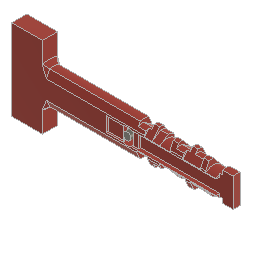
protec3 POC (Autodesk Fusion 360 design; units mm, degrees)
Autodesk Fusion 360 part; units mm, degrees
sketch "base/0 cut" plane through (0, 0, 0) normal (1, 0, 0) x (0, 1, 0)
  line L0 (0, 0) -> (3.3, 0)
  line L1 (3.3, 0) -> (3.3, 3.3)
  circle A0 centre (3.3, 3.3) radius 3.7125
  line L2 (3.3, 3.3) -> (4, 3.3)
  line L3 (3.3, 3.3) -> (2.6, 3.3)
  line L4 (4, 3.3) -> (4, 4.7)
  line L5 (4, 3.3) -> (4, 1.9)
  line L6 (2.6, 3.3) -> (2.6, 1.9)
  line L7 (2.6, 3.3) -> (2.6, 4.7)
  line L8 (4, 4.7) -> (4.775, 4.7)
  line L9 (4, 1.9) -> (4.775, 1.9)
  line L10 (2.6, 1.9) -> (1.825, 1.9)
  line L11 (2.6, 4.7) -> (1.825, 4.7)
  line L12 (4.775, 4.7) -> (4.775, 5.1226)
  line L13 (4.775, 1.9) -> (4.775, 1.4774)
  line L14 (1.825, 1.9) -> (1.825, 1.4774)
  line L15 (1.825, 4.7) -> (1.825, 5.1226)
  line L16 (4.775, 5.1226) -> (4.1363, 6.4923)
  line L17 (4.775, 5.1226) -> (1.825, 5.1226) construction
  line L18 (1.825, 5.1226) -> (2.4637, 6.4923)
  line L19 (1.825, 5.1226) -> (4.775, 5.1226) construction
  arc A1 (4.1363, 6.4923) -> (2.4637, 6.4923) centre (3.3, 3.3) ccw
  line L20 (4.775, 1.4774) -> (4.1363, 0.1077)
  line L21 (4.775, 1.4774) -> (1.825, 1.4774) construction
  line L22 (1.825, 1.4774) -> (2.4637, 0.1077)
  line L23 (1.825, 1.4774) -> (4.775, 1.4774) construction
  arc A2 (2.4637, 0.1077) -> (4.1363, 0.1077) centre (3.3, 3.3) ccw
  dimension "d27" = 3.3
  dimension "d28" = 3.3
  dimension "d29" = 7.425
  dimension "d30" = 0.7
  dimension "d31" = 0.7
  dimension "d32" = 1.4
  dimension "d33" = 1.4
  dimension "d34" = 1.4
  dimension "d35" = 1.4
  dimension "d36" = 0.775
  dimension "d37" = 0.775
  dimension "d38" = 0.775
  dimension "d39" = 0.775
  dimension "d40" = 0.4226
  dimension "d41" = 0.4226
  dimension "d42" = 0.4226
  dimension "d43" = 0.4226
  dimension "d44" = 65
  dimension "d45" = 1.5113
  dimension "d46" = 65
  dimension "d47" = 1.5113
  dimension "d48" = 65
  dimension "d49" = 1.5113
  dimension "d50" = 65
  dimension "d51" = 1.5113
  constraint coincident L0.start origin
  constraint horizontal L0
  constraint perpendicular L0 L1
  constraint coincident L1.end A0.centre
  constraint perpendicular L1 L2
  constraint perpendicular L1 L3
  constraint perpendicular L2 L4
  constraint perpendicular L2 L5
  constraint perpendicular L3 L6
  constraint perpendicular L3 L7
  constraint perpendicular L4 L8
  constraint perpendicular L5 L9
  constraint perpendicular L5 L10
  constraint perpendicular L7 L11
  constraint perpendicular L8 L12
  constraint perpendicular L9 L13
  constraint perpendicular L10 L14
  constraint perpendicular L11 L15
  constraint horizontal L17
  constraint horizontal L19
  constraint horizontal L21
  constraint horizontal L23
  measures "d27" distance of L0.start L0.end
  measures "d28" distance of L0.end L1.end
  measures "d29" diameter of A0
  measures "d30" distance of L1.end L2.end
  measures "d31" distance of L1.end L3.end
  measures "d32" distance of L2.end L4.end
  measures "d33" distance of L2.end L5.end
  measures "d34" distance of L3.end L6.end
  measures "d35" distance of L3.end L7.end
  measures "d36" distance of L4.end L8.end
  measures "d37" distance of L5.end L9.end
  measures "d38" distance of L6.end L10.end
  measures "d39" distance of L7.end L11.end
  measures "d40" distance of L8.end L12.end
  measures "d41" distance of L9.end L13.end
  measures "d42" distance of L10.end L14.end
  measures "d43" distance of L11.end L15.end
  measures "d44" angle of L16 L17
  measures "d45" distance of L12.end L16.end
  measures "d46" angle of L18 L19
  measures "d47" distance of L15.end L18.end
  measures "d48" angle of L20 L21
  measures "d49" distance of L13.end L20.end
  measures "d50" angle of L22 L23
  measures "d51" distance of L14.end L22.end
extrude "Extrude1" add sketch "base/0 cut" against normal blind 42.57 contours L1 L3 L6 L10 L14 L22 A2 | L1 L2 L5 L9 L13 L20 A2 | L2 L3 L4 L7 L8 L11 L12 L15 L16 L18 A1 makes body 1
sketch "bow and bearing retention" plane through (-42.57, 0, 0) normal (-1, 0, 0) x (0, -1, 0)
  line L0 (-2.6, 1.9) -> (-2.6, 4.7)
  line L1 (-2.6, 4.7) -> (-1.825, 4.7)
  line L2 (-1.825, 4.7) -> (-1.825, 5.1226)
  line L3 (-1.825, 5.1226) -> (-2.4637, 6.4923)
  arc A0 (-2.4637, 6.4923) -> (-4.1363, 6.4923) centre (-3.3, 3.3) ccw
  line L4 (-4.1363, 6.4923) -> (-4.775, 5.1226)
  line L5 (-4.775, 5.1226) -> (-4.775, 4.7)
  line L6 (-4.775, 4.7) -> (-4, 4.7)
  line L7 (-4, 4.7) -> (-4, 1.9)
  line L8 (-4, 1.9) -> (-4.775, 1.9)
  line L9 (-4.775, 1.9) -> (-4.775, 1.4774)
  line L10 (-4.775, 1.4774) -> (-4.1363, 0.1077)
  arc A1 (-4.1363, 0.1077) -> (-2.4637, 0.1077) centre (-3.3, 3.3) ccw
  line L11 (-2.4637, 0.1077) -> (-1.825, 1.4774)
  line L12 (-1.825, 1.4774) -> (-1.825, 1.9)
  line L13 (-1.825, 1.9) -> (-2.6, 1.9)
  line L14 (-2.6, 3.3) -> (-3.3, 3.3)
  line L15 (-3.3, 3.3) -> (-3.3, 6.6)
  circle A2 centre (-3.3, 3.3) radius 3.3
  line L16 (-4.775, 4.7) -> (-4.775, 6.252)
  line L17 (-4.775, 6.252) -> (-4.775, 11.252)
  line L18 (-1.825, 4.7) -> (-1.825, 6.252)
  line L19 (-1.825, 6.252) -> (-1.825, 11.252)
  line L20 (-4.775, 11.252) -> (-1.825, 11.252)
  line L21 (-1.825, 1.9) -> (-1.825, 0.348)
  line L22 (-1.825, 0.348) -> (-1.825, -4.652)
  line L23 (-4.775, 1.9) -> (-4.775, 0.348)
  line L24 (-4.775, 0.348) -> (-4.775, -4.652)
  line L25 (-4.775, -4.652) -> (-1.825, -4.652)
  line L26 (-4, 3.3) -> (-4.425, 3.3)
  line L27 (-4.425, 3.3) -> (-4.425, 4.7)
  line L28 (-4.425, 3.3) -> (-4.425, 1.9)
  line L29 (-2.6, 3.3) -> (-2.175, 3.3)
  line L30 (-2.175, 3.3) -> (-2.175, 1.9)
  line L31 (-2.175, 3.3) -> (-2.175, 4.7)
  line L32 (-1.825, 4.7) -> (-1.825, 1.9)
  line L33 (-4.775, 4.7) -> (-4.775, 1.9)
  dimension "d56" = 5
  dimension "d57" = 5
  dimension "d58" = 5
  dimension "d59" = 5
  dimension "d60" = 0.425
  dimension "d61" = 0.425
  constraint midpoint L0 L14.start
  constraint coincident A0.centre A1.centre
  constraint midpoint A0 L15.end
  constraint coincident L15.end A2
  constraint coincident L5.end L6.start
  constraint coincident A2 L16.end
  constraint perpendicular L6 L16
  constraint parallel L16 L17
  constraint coincident L1.end L2.start
  constraint coincident A2 L18.end
  constraint perpendicular L1 L18
  constraint parallel L18 L19
  constraint coincident L12.end L13.start
  constraint coincident A2 L21.end
  constraint perpendicular L13 L21
  constraint parallel L21 L22
  constraint coincident L8.end L9.start
  constraint coincident A2 L23.end
  constraint perpendicular L8 L23
  constraint parallel L23 L24
  constraint midpoint L7 L26.start
  constraint perpendicular L7 L26
  constraint coincident L6 L27.end
  constraint perpendicular L6 L27
  constraint coincident L8 L28.end
  constraint perpendicular L8 L28
  constraint perpendicular L0 L29
  constraint coincident L13 L30.end
  constraint perpendicular L13 L30
  constraint coincident L1 L31.end
  constraint perpendicular L1 L31
  measures "d56" distance of L16.end L17.end
  measures "d57" distance of L18.end L19.end
  measures "d58" distance of L21.end L22.end
  measures "d59" distance of L23.end L24.end
  measures "d60" distance of L26.start L26.end
  measures "d61" distance of L14.start L29.end
extrude "making bearing area wider" add sketch "bow and bearing retention" against normal blind 25.625 contours L0 L13 L29 L30 | L0 L1 L29 L31 | L6 L7 L26 L27 | L7 L8 L26 L28 bodies 1
extrude "making bow" add sketch "bow and bearing retention" against normal blind 6 contours L0 A0 L4 L5 L6 L7 L8 L9 L10 A1 L11 L12 L13 L14 L15 A2 L16 L21 L23 | L0 L13 L29 L30 | L0 L1 L2 L3 A0 L14 L15 A2 L18 | L0 L1 L29 L31 | L1 L13 L30 L31 L32 | A0 A2 L17 L19 L20 | L11 A2 L21 | L3 A2 L18 | L4 A2 L16 | A1 A2 L22 L24 L25 | L10 A2 L23 | L6 L8 L27 L28 L33 | L6 L7 L26 L27 | L7 L8 L26 L28 bodies 1
extrude "strengthening shaft" add 2 faces at (-36.57, 1.9417, 2.8333) (-36.57, 4.5417, 3.7667) along direction (1, 0, 0) blind 12.5 on bodies 1 bodies 1
chamfer "Chamfer1" distance 0.8 angle 45 6 edges at (-36.57, 3.3, 6.6) (-36.57, 2.1443, 5.8074) (-36.57, 4.4557, 5.8074) (-36.57, 4.4557, 0.7926) (-36.57, 3.3, 0) (-36.57, 2.1443, 0.7926) on bodies 1
sketch "tip cut" plane through (0, 0, 0) normal (1, 0, 0) x (0, 1, 0)
  line L0 (0, 0) -> (3.3, 0)
  line L1 (3.3, 0) -> (3.3, 3.3)
  line L2 (3.3, 3.3) -> (2.6, 3.3)
  line L3 (3.3, 3.3) -> (4, 3.3)
  circle A0 centre (3.3, 3.3) radius 2.9
  circle A1 centre (3.3, 3.3) radius 3.3
  line L4 (4, 3.3) -> (4, 0.4858)
  line L5 (4, 3.3) -> (4, 6.1142)
  line L6 (2.6, 3.3) -> (2.6, 0.4858)
  line L7 (2.6, 3.3) -> (2.6, 6.1142)
  dimension "d98" = 3.3
  dimension "d99" = 3.3
  dimension "d100" = 0.7
  dimension "d101" = 0.7
  dimension "d102" = 5.8
  dimension "d103" = 6.6
  constraint coincident L0.start origin
  constraint horizontal L0
  constraint perpendicular L0 L1
  constraint perpendicular L1 L2
  constraint perpendicular L1 L3
  constraint coincident L1.end L2.start
  constraint concentric A0 A1
  constraint coincident A0 L4.end
  constraint perpendicular L3 L4
  constraint coincident A0 L5.end
  constraint perpendicular L3 L5
  constraint coincident A0 L6.end
  constraint perpendicular L2 L6
  constraint coincident A0 L7.end
  constraint perpendicular L2 L7
  measures "d98" distance of L0.start L0.end
  measures "d99" distance of L0.end L1.end
  measures "d100" distance of L1.end L2.end
  measures "d101" distance of L1.end L3.end
  measures "d102" diameter of A0
  measures "d103" diameter of A1
sketch "1 cut" plane through (0, 0, 0) normal (1, 0, 0) x (0, 1, 0)
  line L0 (0, 0) -> (3.3, 0)
  line L1 (3.3, 0) -> (3.3, 3.3)
  line L2 (3.3, 3.3) -> (4, 3.3)
  line L3 (3.3, 3.3) -> (2.6, 3.3)
  line L4 (4, 3.3) -> (4, 4.7)
  line L5 (4, 3.3) -> (4, 1.9)
  line L6 (2.6, 3.3) -> (2.6, 1.9)
  line L7 (2.6, 3.3) -> (2.6, 4.7)
  line L8 (4, 4.7) -> (4.775, 4.7)
  line L9 (4, 1.9) -> (4.775, 1.9)
  line L10 (2.6, 1.9) -> (1.825, 1.9)
  line L11 (2.6, 4.7) -> (1.825, 4.7)
  line L12 (4.775, 4.7) -> (4.775, 4.8422)
  line L13 (1.825, 1.9) -> (1.825, 1.7578)
  line L14 (1.825, 4.7) -> (1.825, 5.1226)
  line L15 (4.775, 1.9) -> (4.775, 1.4774)
  line L16 (1.825, 5.1226) -> (2.4637, 6.4923)
  line L17 (1.825, 5.1226) -> (4.5397, 5.1226) construction
  line L18 (4.775, 1.4774) -> (4.1363, 0.1077)
  line L19 (4.775, 1.4774) -> (2.0603, 1.4774) construction
  line L20 (1.825, 1.7578) -> (3.3, 0)
  line L21 (1.825, 1.7578) -> (4.775, 1.7578) construction
  line L22 (4.775, 4.8422) -> (3.3, 6.6)
  line L23 (4.775, 4.8422) -> (1.825, 4.8422) construction
  arc A0 (3.3, 6.6) -> (2.4637, 6.4923) centre (3.3, 3.3) ccw
  arc A1 (3.3, 0) -> (4.1363, 0.1077) centre (3.3, 3.3) ccw
  circle A2 centre (3.3, 3.3) radius 3.7125
  dimension "d104" = 3.3
  dimension "d105" = 3.3
  dimension "d106" = 0.7
  dimension "d107" = 0.7
  dimension "d108" = 1.4
  dimension "d109" = 1.4
  dimension "d110" = 1.4
  dimension "d111" = 1.4
  dimension "d112" = 0.775
  dimension "d113" = 0.775
  dimension "d114" = 0.775
  dimension "d115" = 0.775
  dimension "d116" = 0.1422
  dimension "d117" = 0.1422
  dimension "d118" = 0.4226
  dimension "d119" = 0.4226
  dimension "d120" = 65
  dimension "d121" = 1.5113
  dimension "d122" = 65
  dimension "d123" = 1.5113
  dimension "d124" = 50
  dimension "d125" = 2.2947
  dimension "d126" = 50
  dimension "d127" = 2.2947
  dimension "d128" = 3.3
  dimension "d129" = 3.3
  dimension "d130" = 7.425
  constraint coincident L0.start origin
  constraint horizontal L0
  constraint perpendicular L0 L1
  constraint perpendicular L1 L2
  constraint perpendicular L1 L3
  constraint perpendicular L2 L4
  constraint perpendicular L2 L5
  constraint perpendicular L3 L6
  constraint perpendicular L3 L7
  constraint perpendicular L4 L8
  constraint perpendicular L5 L9
  constraint perpendicular L6 L10
  constraint perpendicular L7 L11
  constraint perpendicular L8 L12
  constraint perpendicular L10 L13
  constraint perpendicular L11 L14
  constraint perpendicular L9 L15
  constraint horizontal L17
  constraint horizontal L19
  constraint horizontal L21
  constraint horizontal L23
  constraint coincident L14 L23.end
  constraint coincident L17.end L22
  constraint coincident L15 L21.end
  constraint coincident L19.end L20
  constraint concentric A0 A2
  measures "d104" distance of L0.start L0.end
  measures "d105" distance of L0.end L1.end
  measures "d106" distance of L1.end L2.end
  measures "d107" distance of L1.end L3.end
  measures "d108" distance of L2.end L4.end
  measures "d109" distance of L2.end L5.end
  measures "d110" distance of L3.end L6.end
  measures "d111" distance of L3.end L7.end
  measures "d112" distance of L4.end L8.end
  measures "d113" distance of L5.end L9.end
  measures "d114" distance of L6.end L10.end
  measures "d115" distance of L7.end L11.end
  measures "d116" distance of L8.end L12.end
  measures "d117" distance of L10.end L13.end
  measures "d118" distance of L11.end L14.end
  measures "d119" distance of L9.end L15.end
  measures "d120" angle of L16 L17
  measures "d121" distance of L14.end L16.end
  measures "d122" angle of L18 L19
  measures "d123" distance of L15.end L18.end
  measures "d124" angle of L20 L21
  measures "d125" distance of L13.end L0.end
  measures "d126" angle of L22 L23
  measures "d127" distance of L12.end L22.end
  measures "d128" radius of A0
  measures "d129" radius of A1
  measures "d130" diameter of A2
sketch "2 cut" plane through (0, 0, 0) normal (1, 0, 0) x (0, 1, 0)
  line L0 (0, 0) -> (3.3, 0)
  line L1 (3.3, 0) -> (3.3, 3.3)
  line L2 (3.3, 3.3) -> (4, 3.3)
  line L3 (3.3, 3.3) -> (2.6, 3.3)
  line L4 (4, 3.3) -> (4, 4.7)
  line L5 (4, 3.3) -> (4, 1.9)
  line L6 (2.6, 3.3) -> (2.6, 1.9)
  line L7 (2.6, 3.3) -> (2.6, 4.7)
  line L8 (4, 4.7) -> (4.775, 4.7)
  line L9 (4, 1.9) -> (4.775, 1.9)
  line L10 (2.6, 1.9) -> (1.825, 1.9)
  line L11 (2.6, 4.7) -> (1.825, 4.7)
  line L12 (1.825, 4.7) -> (1.825, 4.8422)
  line L13 (4.775, 1.9) -> (4.775, 1.7578)
  line L14 (4.775, 4.7) -> (4.775, 5.1226)
  line L15 (1.825, 1.9) -> (1.825, 1.4774)
  line L16 (1.825, 1.4774) -> (2.4637, 0.1077)
  line L17 (1.825, 1.4774) -> (4.5397, 1.4774) construction
  line L18 (4.775, 5.1226) -> (4.1363, 6.4923)
  line L19 (4.775, 5.1226) -> (2.0603, 5.1226) construction
  line L20 (1.825, 4.8422) -> (3.3, 6.6)
  line L21 (1.825, 4.8422) -> (4.775, 4.8422) construction
  line L22 (4.775, 1.7578) -> (3.3, 0)
  line L23 (4.775, 1.7578) -> (1.825, 1.7578) construction
  arc A0 (2.4637, 0.1077) -> (3.3, 0) centre (3.3, 3.3) ccw
  arc A1 (4.1363, 6.4923) -> (3.3, 6.6) centre (3.3, 3.3) ccw
  circle A2 centre (3.3, 3.3) radius 3.7125
  dimension "d131" = 3.3
  dimension "d132" = 3.3
  dimension "d133" = 0.7
  dimension "d134" = 0.7
  dimension "d135" = 1.4
  dimension "d136" = 1.4
  dimension "d137" = 1.4
  dimension "d138" = 1.4
  dimension "d139" = 0.775
  dimension "d140" = 0.775
  dimension "d141" = 0.775
  dimension "d142" = 0.775
  dimension "d143" = 0.1422
  dimension "d144" = 0.1422
  dimension "d145" = 0.4226
  dimension "d146" = 0.4226
  dimension "d147" = 65
  dimension "d148" = 1.5113
  dimension "d149" = 65
  dimension "d150" = 1.5113
  dimension "d151" = 50
  dimension "d152" = 2.2947
  dimension "d153" = 50
  dimension "d154" = 2.2947
  dimension "d155" = 3.3
  dimension "d156" = 3.3
  dimension "d157" = 7.425
  constraint coincident L0.start origin
  constraint horizontal L0
  constraint perpendicular L0 L1
  constraint perpendicular L1 L2
  constraint perpendicular L1 L3
  constraint perpendicular L2 L4
  constraint perpendicular L2 L5
  constraint perpendicular L3 L6
  constraint perpendicular L3 L7
  constraint perpendicular L4 L8
  constraint perpendicular L5 L9
  constraint perpendicular L6 L10
  constraint perpendicular L7 L11
  constraint perpendicular L11 L12
  constraint perpendicular L9 L13
  constraint perpendicular L8 L14
  constraint perpendicular L10 L15
  constraint horizontal L17
  constraint horizontal L19
  constraint horizontal L21
  constraint horizontal L23
  constraint concentric A1 A2
  constraint coincident L15 L23.end
  constraint coincident L17.end L22
  constraint coincident L14 L21.end
  constraint coincident L19.end L20
  measures "d131" distance of L0.start L0.end
  measures "d132" distance of L0.end L1.end
  measures "d133" distance of L1.end L2.end
  measures "d134" distance of L1.end L3.end
  measures "d135" distance of L2.end L4.end
  measures "d136" distance of L2.end L5.end
  measures "d137" distance of L3.end L6.end
  measures "d138" distance of L3.end L7.end
  measures "d139" distance of L4.end L8.end
  measures "d140" distance of L5.end L9.end
  measures "d141" distance of L6.end L10.end
  measures "d142" distance of L7.end L11.end
  measures "d143" distance of L11.end L12.end
  measures "d144" distance of L9.end L13.end
  measures "d145" distance of L8.end L14.end
  measures "d146" distance of L10.end L15.end
  measures "d147" angle of L16 L17
  measures "d148" distance of L15.end L16.end
  measures "d149" angle of L18 L19
  measures "d150" distance of L14.end L18.end
  measures "d151" angle of L20 L21
  measures "d152" distance of L12.end L20.end
  measures "d153" angle of L22 L23
  measures "d154" distance of L13.end L0.end
  measures "d155" radius of A0
  measures "d156" radius of A1
  measures "d157" diameter of A2
sketch "3 cut" plane through (0, 0, 0) normal (1, 0, 0) x (0, 1, 0)
  line L0 (0, 0) -> (3.3, 0)
  line L1 (3.3, 0) -> (3.3, 3.3)
  line L2 (3.3, 3.3) -> (4, 3.3)
  line L3 (3.3, 3.3) -> (2.6, 3.3)
  line L4 (4, 3.3) -> (4, 4.7)
  line L5 (4, 3.3) -> (4, 1.9)
  line L6 (2.6, 3.3) -> (2.6, 1.9)
  line L7 (2.6, 3.3) -> (2.6, 4.7)
  line L8 (4, 4.7) -> (4.775, 4.7)
  line L9 (4, 1.9) -> (4.775, 1.9)
  line L10 (2.6, 1.9) -> (1.825, 1.9)
  line L11 (2.6, 4.7) -> (1.825, 4.7)
  line L12 (4.775, 4.7) -> (4.775, 4.8422)
  line L13 (1.825, 1.9) -> (1.825, 1.7578)
  line L14 (1.825, 4.7) -> (1.825, 5.1226)
  line L15 (4.775, 1.9) -> (4.775, 1.4774)
  line L16 (4.775, 1.4774) -> (4.4962, 0.8794)
  line L17 (4.775, 1.4774) -> (2.2255, 1.4774) construction
  line L18 (1.825, 5.1226) -> (2.1038, 5.7206)
  line L19 (1.825, 5.1226) -> (4.3745, 5.1226) construction
  line L20 (4.775, 4.8422) -> (3.1292, 5.9946)
  line L21 (4.775, 4.8422) -> (1.825, 4.8422) construction
  line L22 (1.825, 1.7578) -> (3.4708, 0.6054)
  line L23 (1.825, 1.7578) -> (4.775, 1.7578) construction
  arc A0 (3.1292, 5.9946) -> (2.1038, 5.7206) centre (3.3, 3.3) ccw
  arc A1 (3.4708, 0.6054) -> (4.4962, 0.8794) centre (3.3, 3.3) ccw
  circle A2 centre (3.3, 3.3) radius 3.7125
  dimension "d158" = 3.3
  dimension "d159" = 3.3
  dimension "d160" = 0.7
  dimension "d161" = 0.7
  dimension "d162" = 1.4
  dimension "d163" = 1.4
  dimension "d164" = 1.4
  dimension "d165" = 1.4
  dimension "d166" = 0.775
  dimension "d167" = 0.775
  dimension "d168" = 0.775
  dimension "d169" = 0.775
  dimension "d170" = 0.1422
  dimension "d171" = 0.1422
  dimension "d172" = 0.4226
  dimension "d173" = 0.4226
  dimension "d174" = 65
  dimension "d175" = 0.6598
  dimension "d176" = 65
  dimension "d177" = 0.6598
  dimension "d178" = 35
  dimension "d179" = 2.0092
  dimension "d180" = 35
  dimension "d181" = 2.0092
  dimension "d182" = 2.7
  dimension "d183" = 2.7
  dimension "d184" = 7.425
  constraint coincident L0.start origin
  constraint horizontal L0
  constraint perpendicular L0 L1
  constraint perpendicular L1 L2
  constraint perpendicular L1 L3
  constraint perpendicular L2 L4
  constraint perpendicular L2 L5
  constraint perpendicular L3 L6
  constraint perpendicular L3 L7
  constraint perpendicular L4 L8
  constraint perpendicular L5 L9
  constraint perpendicular L6 L10
  constraint perpendicular L7 L11
  constraint perpendicular L8 L12
  constraint perpendicular L10 L13
  constraint perpendicular L11 L14
  constraint perpendicular L9 L15
  constraint horizontal L17
  constraint horizontal L19
  constraint horizontal L21
  constraint horizontal L23
  constraint coincident L17.end L22
  constraint coincident L14 L21.end
  constraint coincident L19.end L20
  constraint coincident L15 L23.end
  constraint concentric A0 A2
  measures "d158" distance of L0.start L0.end
  measures "d159" distance of L0.end L1.end
  measures "d160" distance of L1.end L2.end
  measures "d161" distance of L1.end L3.end
  measures "d162" distance of L2.end L4.end
  measures "d163" distance of L2.end L5.end
  measures "d164" distance of L3.end L6.end
  measures "d165" distance of L3.end L7.end
  measures "d166" distance of L4.end L8.end
  measures "d167" distance of L5.end L9.end
  measures "d168" distance of L6.end L10.end
  measures "d169" distance of L7.end L11.end
  measures "d170" distance of L8.end L12.end
  measures "d171" distance of L10.end L13.end
  measures "d172" distance of L11.end L14.end
  measures "d173" distance of L9.end L15.end
  measures "d174" angle of L16 L17
  measures "d175" distance of L15.end L16.end
  measures "d176" angle of L18 L19
  measures "d177" distance of L14.end L18.end
  measures "d178" angle of L20 L21
  measures "d179" distance of L12.end L20.end
  measures "d180" angle of L22 L23
  measures "d181" distance of L13.end L22.end
  measures "d182" radius of A0
  measures "d183" radius of A1
  measures "d184" diameter of A2
sketch "4 cut" plane through (0, 0, 0) normal (1, 0, 0) x (0, 1, 0)
  line L0 (0, 0) -> (3.3, 0)
  line L1 (3.3, 0) -> (3.3, 3.3)
  line L2 (3.3, 3.3) -> (4, 3.3)
  line L3 (3.3, 3.3) -> (2.6, 3.3)
  line L4 (4, 3.3) -> (4, 1.9)
  line L5 (4, 3.3) -> (4, 4.7)
  line L6 (2.6, 3.3) -> (2.6, 1.9)
  line L7 (2.6, 3.3) -> (2.6, 4.7)
  line L8 (4, 4.7) -> (4.775, 4.7)
  line L9 (4, 1.9) -> (4.775, 1.9)
  line L10 (2.6, 1.9) -> (1.825, 1.9)
  line L11 (2.6, 4.7) -> (1.825, 4.7)
  line L12 (4.775, 4.7) -> (4.775, 4.8422)
  line L13 (1.825, 4.7) -> (1.825, 4.8422)
  line L14 (4.775, 1.9) -> (4.775, 1.7578)
  line L15 (1.825, 1.9) -> (1.825, 1.7578)
  line L16 (4.775, 4.8422) -> (3.8512, 5.9431)
  line L17 (4.775, 4.8422) -> (1.825, 4.8422) construction
  line L18 (1.825, 4.8422) -> (2.7488, 5.9431)
  line L19 (1.825, 4.8422) -> (4.775, 4.8422) construction
  line L20 (4.775, 1.7578) -> (3.8512, 0.6569)
  line L21 (4.775, 1.7578) -> (1.825, 1.7578) construction
  line L22 (1.825, 1.7578) -> (2.7488, 0.6569)
  line L23 (1.825, 1.7578) -> (4.775, 1.7578) construction
  arc A0 (3.8512, 5.9431) -> (2.7488, 5.9431) centre (3.3, 3.3) ccw
  arc A1 (2.7488, 0.6569) -> (3.8512, 0.6569) centre (3.3, 3.3) ccw
  circle A2 centre (3.3, 3.3) radius 3.7125
  dimension "d185" = 3.3
  dimension "d186" = 3.3
  dimension "d187" = 0.7
  dimension "d188" = 0.7
  dimension "d189" = 1.4
  dimension "d190" = 1.4
  dimension "d191" = 1.4
  dimension "d192" = 1.4
  dimension "d193" = 0.775
  dimension "d194" = 0.775
  dimension "d195" = 0.775
  dimension "d196" = 0.775
  dimension "d197" = 0.1422
  dimension "d198" = 0.1422
  dimension "d199" = 0.1422
  dimension "d200" = 0.1422
  dimension "d201" = 50
  dimension "d202" = 1.4372
  dimension "d203" = 50
  dimension "d204" = 1.4372
  dimension "d205" = 50
  dimension "d206" = 1.4372
  dimension "d207" = 50
  dimension "d208" = 1.4372
  dimension "d209" = 7.425
  constraint coincident L0.start origin
  constraint horizontal L0
  constraint perpendicular L0 L1
  constraint perpendicular L1 L2
  constraint perpendicular L1 L3
  constraint perpendicular L3 L4
  constraint perpendicular L2 L5
  constraint perpendicular L3 L6
  constraint perpendicular L3 L7
  constraint perpendicular L5 L8
  constraint perpendicular L4 L9
  constraint perpendicular L6 L10
  constraint perpendicular L7 L11
  constraint perpendicular L8 L12
  constraint perpendicular L11 L13
  constraint perpendicular L9 L14
  constraint perpendicular L10 L15
  constraint horizontal L17
  constraint horizontal L19
  constraint horizontal L21
  constraint horizontal L23
  constraint coincident L1.end L2.start
  constraint concentric A0 A2
  measures "d185" distance of L0.start L0.end
  measures "d186" distance of L0.end L1.end
  measures "d187" distance of L1.end L2.end
  measures "d188" distance of L1.end L3.end
  measures "d189" distance of L2.end L4.end
  measures "d190" distance of L2.end L5.end
  measures "d191" distance of L3.end L6.end
  measures "d192" distance of L3.end L7.end
  measures "d193" distance of L5.end L8.end
  measures "d194" distance of L4.end L9.end
  measures "d195" distance of L6.end L10.end
  measures "d196" distance of L7.end L11.end
  measures "d197" distance of L8.end L12.end
  measures "d198" distance of L11.end L13.end
  measures "d199" distance of L9.end L14.end
  measures "d200" distance of L10.end L15.end
  measures "d201" angle of L16 L17
  measures "d202" distance of L12.end L16.end
  measures "d203" angle of L18 L19
  measures "d204" distance of L13.end L18.end
  measures "d205" angle of L20 L21
  measures "d206" distance of L14.end L20.end
  measures "d207" angle of L22 L23
  measures "d208" distance of L15.end L22.end
  measures "d209" diameter of A2
sketch "5 cut" plane through (0, 0, 0) normal (1, 0, 0) x (0, 1, 0)
  line L0 (0, 0) -> (3.3, 0)
  line L1 (3.3, 0) -> (3.3, 3.3)
  line L2 (3.3, 3.3) -> (4, 3.3)
  line L3 (3.3, 3.3) -> (2.6, 3.3)
  line L4 (4, 3.3) -> (4, 4.7)
  line L5 (4, 3.3) -> (4, 1.9)
  line L6 (2.6, 3.3) -> (2.6, 1.9)
  line L7 (2.6, 3.3) -> (2.6, 4.7)
  line L8 (4, 4.7) -> (4.775, 4.7)
  line L9 (4, 1.9) -> (4.775, 1.9)
  line L10 (2.6, 1.9) -> (1.825, 1.9)
  line L11 (2.6, 4.7) -> (1.825, 4.7)
  line L12 (1.825, 4.7) -> (1.825, 4.8422)
  line L13 (4.775, 1.9) -> (4.775, 1.7578)
  line L14 (1.825, 1.9) -> (1.825, 1.4774)
  line L15 (4.775, 4.7) -> (4.775, 5.1226)
  line L16 (1.825, 4.8422) -> (3.4708, 5.9946)
  line L17 (1.825, 4.8422) -> (4.775, 4.8422) construction
  line L18 (4.775, 1.7578) -> (3.1292, 0.6054)
  line L19 (4.775, 1.7578) -> (1.825, 1.7578) construction
  line L20 (1.825, 1.4774) -> (2.1038, 0.8794)
  line L21 (1.825, 1.4774) -> (4.3745, 1.4774) construction
  line L22 (4.775, 5.1226) -> (4.4962, 5.7206)
  line L23 (4.775, 5.1226) -> (2.2255, 5.1226) construction
  arc A0 (4.4962, 5.7206) -> (3.4708, 5.9946) centre (3.3, 3.3) ccw
  arc A1 (2.1038, 0.8794) -> (3.1292, 0.6054) centre (3.3, 3.3) ccw
  circle A2 centre (3.3, 3.3) radius 3.7125
  dimension "d210" = 3.3
  dimension "d211" = 3.3
  dimension "d212" = 0.7
  dimension "d213" = 0.7
  dimension "d214" = 1.4
  dimension "d215" = 1.4
  dimension "d216" = 1.4
  dimension "d217" = 1.4
  dimension "d218" = 0.775
  dimension "d219" = 0.775
  dimension "d220" = 0.775
  dimension "d221" = 0.775
  dimension "d222" = 0.1422
  dimension "d223" = 0.1422
  dimension "d224" = 0.4226
  dimension "d225" = 0.4226
  dimension "d226" = 35
  dimension "d227" = 2.0092
  dimension "d228" = 35
  dimension "d229" = 2.0092
  dimension "d230" = 0.6598
  dimension "d231" = 65
  dimension "d232" = 65
  dimension "d233" = 0.6598
  dimension "d234" = 2.7
  dimension "d235" = 2.7
  dimension "d236" = 7.425
  constraint coincident L0.start origin
  constraint horizontal L0
  constraint perpendicular L0 L1
  constraint perpendicular L1 L2
  constraint perpendicular L1 L3
  constraint perpendicular L2 L4
  constraint perpendicular L2 L5
  constraint perpendicular L3 L6
  constraint perpendicular L3 L7
  constraint perpendicular L4 L8
  constraint perpendicular L5 L9
  constraint perpendicular L6 L10
  constraint perpendicular L7 L11
  constraint perpendicular L11 L12
  constraint perpendicular L9 L13
  constraint perpendicular L10 L14
  constraint perpendicular L8 L15
  constraint horizontal L17
  constraint horizontal L19
  constraint horizontal L21
  constraint horizontal L23
  constraint concentric A0 A2
  constraint coincident L14 L19.end
  constraint coincident L18 L21.end
  constraint coincident L15 L17.end
  constraint coincident L16 L23.end
  measures "d210" distance of L0.start L0.end
  measures "d211" distance of L0.end L1.end
  measures "d212" distance of L1.end L2.end
  measures "d213" distance of L1.end L3.end
  measures "d214" distance of L2.end L4.end
  measures "d215" distance of L2.end L5.end
  measures "d216" distance of L3.end L6.end
  measures "d217" distance of L3.end L7.end
  measures "d218" distance of L4.end L8.end
  measures "d219" distance of L5.end L9.end
  measures "d220" distance of L6.end L10.end
  measures "d221" distance of L7.end L11.end
  measures "d222" distance of L11.end L12.end
  measures "d223" distance of L9.end L13.end
  measures "d224" distance of L10.end L14.end
  measures "d225" distance of L8.end L15.end
  measures "d226" angle of L16 L17
  measures "d227" distance of L12.end L16.end
  measures "d228" angle of L18 L19
  measures "d229" distance of L13.end L18.end
  measures "d230" distance of L14.end L20.end
  measures "d231" angle of L20 L21
  measures "d232" angle of L22 L23
  measures "d233" distance of L15.end L22.end
  measures "d234" radius of A0
  measures "d235" radius of A1
  measures "d236" diameter of A2
sketch "6 cut" plane through (0, 0, 0) normal (1, 0, 0) x (0, 1, 0)
  line L0 (0, 0) -> (3.3, 0)
  line L1 (3.3, 0) -> (3.3, 3.3)
  line L2 (3.3, 3.3) -> (4, 3.3)
  line L3 (4, 3.3) -> (4, 4.7)
  line L4 (4, 4.7) -> (4.775, 4.7)
  line L5 (4.775, 4.7) -> (4.775, 4.8422)
  line L6 (4.775, 4.8422) -> (3.1292, 5.9946) construction
  line L7 (4.775, 4.8422) -> (1.861, 4.8422) construction
  circle A0 centre (3.3, 3.3) radius 2.1093
  circle A1 centre (3.3, 3.3) radius 3.7125
  dimension "d237" = 3.3
  dimension "d238" = 3.3
  dimension "d239" = 0.7
  dimension "d240" = 1.4
  dimension "d241" = 0.775
  dimension "d242" = 0.1422
  dimension "d243" = 35
  dimension "d244" = 2.0092
  dimension "d245" = 7.425
  constraint coincident L0.start origin
  constraint horizontal L0
  constraint perpendicular L0 L1
  constraint perpendicular L1 L2
  constraint perpendicular L2 L3
  constraint perpendicular L3 L4
  constraint perpendicular L4 L5
  constraint horizontal L7
  constraint coincident L1.end L2.start
  constraint tangent L6 A0
  constraint coincident L7.end A0
  constraint concentric A0 A1
  measures "d237" distance of L0.start L0.end
  measures "d238" distance of L0.end L1.end
  measures "d239" distance of L1.end L2.end
  measures "d240" distance of L2.end L3.end
  measures "d241" distance of L3.end L4.end
  measures "d242" distance of L4.end L5.end
  measures "d243" angle of L6 L7
  measures "d244" distance of L5.end L6.end
  measures "d245" diameter of A1
extrude "tip" cut sketch "tip cut" against normal blind 2.57 contours A0 L6 L7 | A0 L4 L5 | A1 bodies 1
extrude "0" cut sketch "6 cut" along normal mid plane 1 from surface at -2.57 bodies 1
extrude "1" cut sketch "6 cut" along normal mid plane 2 from surface at -3.57 bodies 1
extrude "2" cut sketch "1 cut" along normal mid plane 2 from surface at -5.07 bodies 1
extrude "3" cut sketch "4 cut" along normal mid plane 2 from surface at -6.57 bodies 1
extrude "4" cut sketch "2 cut" along normal mid plane 2 from surface at -8.07 bodies 1
extrude "5" cut sketch "3 cut" along normal mid plane 2 from surface at -9.57 bodies 1
extrude "6" cut sketch "1 cut" along normal mid plane 2 from surface at -11.07 bodies 1
extrude "7" cut sketch "6 cut" along normal mid plane 2 from surface at -12.57 bodies 1
extrude "8" cut sketch "5 cut" along normal mid plane 2 from surface at -14.07 bodies 1
extrude "9" cut sketch "2 cut" along normal mid plane 2 from surface at -15.57 bodies 1
extrude "10" cut sketch "3 cut" along normal mid plane 2 from surface at -17.07 bodies 1
sketch "dc bearing hole" plane through (0, 2.6, 0) normal (0, -1, 0) x (1, 0, 0)
  line L0 (0, 0.4858) -> (0, 6.1142)
  line L1 (-2.57, 4.7) -> (-18.07, 4.7)
  line L2 (-18.07, 1.9) -> (-2.57, 1.9)
  line L3 (0, 3.3) -> (-20, 3.3)
  circle A0 centre (-20, 3.3) radius 1.6
  line L4 (-2.57, 1.9) -> (-2.57, 1.3102)
  line L5 (-2.57, 1.3102) -> (-2.07, 1.3102)
  line L6 (-2.07, 1.3102) -> (-2.07, 0.4858)
  line L7 (-2.07, 0.4858) -> (0, 0.4858)
  line L8 (0, 6.1142) -> (-2.07, 6.1142)
  line L9 (-2.07, 6.1142) -> (-2.07, 5.2898)
  line L10 (-2.07, 5.2898) -> (-2.57, 5.2898)
  line L11 (-2.57, 5.2898) -> (-2.57, 4.7)
  line L12 (-18.07, 4.7) -> (-18.07, 1.9)
  dimension "d54" = 20
  dimension "d55" = 3.2
  constraint midpoint L0 L3.start
  constraint perpendicular L0 L3
  constraint coincident L3.end A0.centre
  measures "d54" distance of L3.start L3.end
  measures "d55" diameter of A0
extrude "Extrude22" cut sketch "dc bearing hole" along normal mid plane 15 contours A0 bodies 1
ref_plane "WorkPlane2" through (-20, 3.3, 3.3) normal (0, -1, 0) x (1, 0, 0)
sketch "Sketch14" plane through (0, 3.3, 0) normal (0, -1, 0) x (-1, 0, 0)
  line L0 (0, 0) -> (0, -3.3) construction
  line L1 (0, -3.3) -> (20, -3.3) construction
  circle A0 centre (20, -3.3) radius 0.75
  circle A1 centre (20, -3.3) radius 1.6 construction
  line L2 (18.4, -3.3) -> (19.25, -3.3) construction
  circle A2 centre (20, -3.3) radius 1
  line L3 (19.25, -3.3) -> (19.05, -3.3) construction
  line L4 (19.05, -3.3) -> (19.05, -4.5874)
  line L5 (19.05, -3.3) -> (19.05, -2.0126)
  line L6 (20, -3.3) -> (20.75, -3.3) construction
  line L7 (20.75, -3.3) -> (20.95, -3.3) construction
  line L8 (20.95, -3.3) -> (20.95, -4.5874)
  line L9 (20.95, -3.3) -> (20.95, -2.0126)
  arc A3 (20.95, -4.5874) -> (20.95, -2.0126) centre (20, -3.3) ccw
  arc A4 (19.05, -2.0126) -> (19.05, -4.5874) centre (20, -3.3) ccw
  dimension "d282" = 3.3
  dimension "d283" = 20
  dimension "d286" = 1.5
  dimension "d289" = 3.2
  dimension "d290" = 2
  dimension "d291" = 0.2
  dimension "d292" = 0.2
  constraint coincident L0.start origin
  constraint vertical L0
  constraint perpendicular L0 L1
  constraint coincident L1.end A0.centre
  constraint concentric A0 A1
  constraint coincident A1 L2.start
  constraint coincident L1 L2.start
  constraint coincident A0 L2.end
  constraint coincident L1 L2.end
  constraint concentric A1 A2
  constraint parallel L2 L3
  constraint coincident A1 L4.end
  constraint perpendicular L3 L4
  constraint coincident A1 L5.end
  constraint perpendicular L3 L5
  constraint coincident A0 L6.end
  constraint parallel L1 L6
  constraint parallel L6 L7
  constraint coincident A1 L8.end
  constraint perpendicular L7 L8
  constraint coincident A1 L9.end
  constraint perpendicular L7 L9
  measures "d282" distance of L0.start L0.end
  measures "d283" distance of L0.end L1.end
  measures "d286" diameter of A0
  measures "d289" diameter of A1
  measures "d290" diameter of A2
  measures "d291" distance of L2.end L3.end
  measures "d292" distance of L6.end L7.end
extrude "Extrude23" add sketch "Sketch14" along normal mid plane 2.95 separate body contours A0 makes body 2
extrude "Extrude24" add sketch "Sketch14" along normal mid plane 0.5 contours A2 L8 L9 | A2 L4 L5 L8 L9 | A2 L4 L5 bodies 2
extrude "Extrude25" add sketch "Sketch14" against normal blind 0.7 from surface at 1.125 contours A2 L8 L9 | A2 L8 L9 A3 | A2 L4 L5 | A2 L4 L5 A4 bodies 1
extrude "Extrude26" add sketch "Sketch14" along normal blind 0.7 from surface at -1.125 contours A2 L8 L9 | A2 L8 L9 A3 | A2 L4 L5 | A2 L4 L5 A4 bodies 1
equation "key_width = 2.95 mm"
equation "half_key_width = 0.5 * key_width"
equation "radius_one = 3.3 mm"
equation "radius_two = 2.7 mm"
equation "zero_disk_angle = 65 deg"
equation "one_two_disk_angle = zero_disk_angle - 15 deg"
equation "three_five_disk_angle = one_two_disk_angle - 15 deg"
equation "uncut_diagonal_width = 4.25 mm"
equation "half_key_side_height = ( 0.5 * 2.8 ) * 1 mm"
equation "zero_disk_height_full = 0.5 * ( ( ( ( uncut_diagonal_width / cos(90 deg - zero_disk_angle) ) ^ 2 ) - ( key_width ^ 2 ) ) ^ 0.5 )"
equation "zero_disk_height_partial = zero_disk_height_full - half_key_side_height"
equation "cut_height_full = ( radius_one ) - ( half_key_width / tan(40 deg) )"
equation "cut_height_partial = cut_height_full - half_key_side_height"
equation "a = -half_key_width"
equation "b1 = zero_disk_height_full"
equation "b2 = cut_height_full"
equation "x1 = ( -2 * tan(zero_disk_angle) * ( b1 - a * tan(zero_disk_angle) ) + sqrt(( 2 * tan(zero_disk_angle) * ( b1 - a * tan(zero_disk_angle) ) ) ^ 2 - 4 * ( 1 + ( tan(zero_disk_angle) ) ^ 2 ) * ( ( b1 - a * tan(zero_disk_angle) ) ^ 2 - radius_one ^ 2 )) ) / ( 2 * ( 1 + ( tan(zero_disk_angle) ) ^ 2 ) )"
equation "zero_cut_side_height = sqrt(( x1 - a ) ^ 2 + ( x1 * tan(zero_disk_angle) + b1 - a * tan(zero_disk_angle) - b1 ) ^ 2)"
equation "x2 = ( -2 * tan(three_five_disk_angle) * ( b2 - a * tan(three_five_disk_angle) ) + sqrt(( 2 * tan(three_five_disk_angle) * ( b2 - a * tan(three_five_disk_angle) ) ) ^ 2 - 4 * ( 1 + ( tan(three_five_disk_angle) ) ^ 2 ) * ( ( b2 - a * tan(three_five_disk_angle) ) ^ 2 - radius_two ^ 2 )) ) / ( 2 * ( 1 + ( tan(three_five_disk_angle) ) ^ 2 ) )"
equation "three_five_cut_side_height = sqrt(( x2 - a ) ^ 2 + ( x2 * tan(three_five_disk_angle) + b2 - a * tan(three_five_disk_angle) - b2 ) ^ 2)"
equation "x3 = ( -2 * tan(one_two_disk_angle) * ( b2 - a * tan(one_two_disk_angle) ) + sqrt(( 2 * tan(one_two_disk_angle) * ( b2 - a * tan(one_two_disk_angle) ) ) ^ 2 - 4 * ( 1 + ( tan(one_two_disk_angle) ) ^ 2 ) * ( ( b2 - a * tan(one_two_disk_angle) ) ^ 2 - radius_two ^ 2 )) ) / ( 2 * ( 1 + ( tan(one_two_disk_angle) ) ^ 2 ) )"
equation "four_cut_side_height = sqrt(( x3 - a ) ^ 2 + ( x3 * tan(one_two_disk_angle) + b2 - a * tan(one_two_disk_angle) - b2 ) ^ 2)"
equation "x4 = ( -2 * tan(one_two_disk_angle) * ( b2 - a * tan(one_two_disk_angle) ) + sqrt(( 2 * tan(one_two_disk_angle) * ( b2 - a * tan(one_two_disk_angle) ) ) ^ 2 - 4 * ( 1 + ( tan(one_two_disk_angle) ) ^ 2 ) * ( ( b2 - a * tan(one_two_disk_angle) ) ^ 2 - radius_one ^ 2 )) ) / ( 2 * ( 1 + ( tan(one_two_disk_angle) ) ^ 2 ) )"
equation "one_two_cut_side_height = sqrt(( x4 - a ) ^ 2 + ( x4 * tan(one_two_disk_angle) + b2 - a * tan(one_two_disk_angle) - b2 ) ^ 2)"
equation "x5 = ( -2 * tan(zero_disk_angle) * ( b1 - a * tan(zero_disk_angle) ) + sqrt(( 2 * tan(zero_disk_angle) * ( b1 - a * tan(zero_disk_angle) ) ) ^ 2 - 4 * ( 1 + ( tan(zero_disk_angle) ) ^ 2 ) * ( ( b1 - a * tan(zero_disk_angle) ) ^ 2 - radius_two ^ 2 )) ) / ( 2 * ( 1 + ( tan(zero_disk_angle) ) ^ 2 ) )"
equation "zero_cut_three_five_side_height = sqrt(( x5 - a ) ^ 2 + ( x5 * tan(zero_disk_angle) + b1 - a * tan(zero_disk_angle) - b1 ) ^ 2)"
equation "d27 = radius_one"
equation "d28 = d27"
equation "d29 = 2.25 * radius_one"
equation "d30 = half_key_width - 0.775 mm"
equation "d31 = d30"
equation "d32 = half_key_side_height"
equation "d33 = d32"
equation "d34 = d32"
equation "d35 = d32"
equation "d36 = half_key_width - d30"
equation "d37 = d36"
equation "d38 = d36"
equation "d39 = d36"
equation "d40 = zero_disk_height_partial"
equation "d41 = d40"
equation "d42 = d40"
equation "d43 = d40"
equation "d44 = zero_disk_angle"
equation "d45 = zero_cut_side_height"
equation "d46 = d44"
equation "d47 = d45"
equation "d48 = d44"
equation "d49 = d45"
equation "d50 = d44"
equation "d51 = d45"
equation "d52 = -( 2.57 mm + 35 mm + 2 mm + 3 mm )"
equation "d57 = d56"
equation "d58 = d56"
equation "d59 = d56"
equation "d61 = d60"
equation "d62 = -16.8 mm - 1.375 mm - 0.1 mm - 0.35 mm - 2 mm - 3 mm - 2 mm"
equation "d66 = 13.5 mm - 6 mm + 2 mm + 3 mm"
equation "d98 = radius_one"
equation "d99 = radius_one"
equation "d100 = d30"
equation "d101 = d30"
equation "d103 = 2 * radius_one"
equation "d104 = radius_one"
equation "d105 = radius_one"
equation "d106 = d30"
equation "d107 = d30"
equation "d108 = d32"
equation "d109 = d32"
equation "d110 = d32"
equation "d111 = d32"
equation "d112 = d36"
equation "d113 = d36"
equation "d114 = d36"
equation "d115 = d36"
equation "d116 = cut_height_partial"
equation "d117 = d116"
equation "d118 = d40"
equation "d119 = d40"
equation "d120 = d44"
equation "d121 = d45"
equation "d122 = d44"
equation "d123 = d45"
equation "d124 = one_two_disk_angle"
equation "d125 = one_two_cut_side_height"
equation "d126 = d124"
equation "d127 = d125"
equation "d130 = d29"
equation "d131 = radius_one"
equation "d132 = radius_one"
equation "d133 = d30"
equation "d134 = d30"
equation "d135 = d32"
equation "d136 = d32"
equation "d137 = d32"
equation "d138 = d32"
equation "d139 = d36"
equation "d140 = d36"
equation "d141 = d36"
equation "d142 = d36"
equation "d143 = d116"
equation "d144 = d116"
equation "d145 = d40"
equation "d146 = d40"
equation "d147 = d44"
equation "d148 = d45"
equation "d149 = d44"
equation "d150 = d45"
equation "d151 = d124"
equation "d152 = d125"
equation "d153 = d124"
equation "d154 = d125"
equation "d157 = d29"
equation "d158 = radius_one"
equation "d159 = radius_one"
equation "d160 = d30"
equation "d161 = d30"
equation "d162 = d32"
equation "d163 = d32"
equation "d164 = d32"
equation "d165 = d32"
equation "d166 = d36"
equation "d167 = d36"
equation "d168 = d36"
equation "d169 = d36"
equation "d170 = d116"
equation "d171 = d116"
equation "d172 = d40"
equation "d173 = d40"
equation "d174 = d44"
equation "d175 = zero_cut_three_five_side_height"
equation "d176 = d44"
equation "d177 = d175"
equation "d178 = three_five_disk_angle"
equation "d179 = three_five_cut_side_height"
equation "d180 = d178"
equation "d181 = d179"
equation "d184 = d29"
equation "d185 = radius_one"
equation "d186 = radius_one"
equation "d187 = d30"
equation "d188 = d30"
equation "d189 = d32"
equation "d190 = d32"
equation "d191 = d32"
equation "d192 = d32"
equation "d193 = d36"
equation "d194 = d36"
equation "d195 = d36"
equation "d196 = d36"
equation "d197 = d116"
equation "d198 = d116"
equation "d199 = d116"
equation "d200 = d116"
equation "d201 = d124"
equation "d202 = four_cut_side_height"
equation "d203 = d124"
equation "d204 = d202"
equation "d205 = d124"
equation "d206 = d202"
equation "d207 = d124"
equation "d208 = d202"
equation "d209 = d29"
equation "d210 = radius_one"
equation "d211 = radius_one"
equation "d212 = d30"
equation "d213 = d30"
equation "d214 = d32"
equation "d215 = d32"
equation "d216 = d32"
equation "d217 = d32"
equation "d218 = d36"
equation "d219 = d36"
equation "d220 = d36"
equation "d221 = d36"
equation "d222 = d116"
equation "d223 = d116"
equation "d224 = d40"
equation "d225 = d40"
equation "d226 = d178"
equation "d227 = d179"
equation "d228 = d178"
equation "d229 = d179"
equation "d230 = d175"
equation "d231 = d44"
equation "d232 = d44"
equation "d233 = d175"
equation "d236 = d29"
equation "d237 = radius_one"
equation "d238 = radius_one"
equation "d239 = d30"
equation "d240 = d32"
equation "d241 = d36"
equation "d242 = d116"
equation "d243 = d178"
equation "d244 = d179"
equation "d245 = d29"
equation "d251 = -2.07 mm - ( 1.5 * 1 mm )"
equation "d254 = -2.07 mm - ( 1.5 * 2 mm )"
equation "d257 = -2.07 mm - ( 1.5 * 3 mm )"
equation "d260 = -2.07 mm - ( 1.5 * 4 mm )"
equation "d263 = -2.07 mm - ( 1.5 * 5 mm )"
equation "d266 = -2.07 mm - ( 1.5 * 6 mm )"
equation "d269 = -2.07 mm - ( 1.5 * 7 mm )"
equation "d272 = -2.07 mm - ( 1.5 * 8 mm )"
equation "d275 = -2.07 mm - ( 1.5 * 9 mm )"
equation "d278 = -2.07 mm - ( 1.5 * 10 mm )"
equation "d282 = radius_one"
equation "d283 = d54"
equation "d287 = half_key_width"
equation "d292 = d291"
named bodies: "blade"
